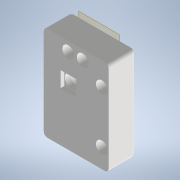
# Autodesk Inventor part: 30_ESP32_Camera_tray
Saved by Autodesk Inventor 2022 (Build 260153000, 153)
## iProperties
Created: 2022-06-11
Part Number: 30_ESP32_Camera_tray
Material: Generisch
Document SubType Name: Modeling
Designer: diederichbenedict
Density: 1 g/cm^3
Appearance: Vorgabe
Author: diederichbenedict
Autodesk Inventor part; units mm, degrees
ref_plane "YZ Plane" through (0, 0, 0) normal (1, 0, 0) x (0, 1, 0)
ref_plane "XZ Plane" through (0, 0, 0) normal (0, 1, 0) x (-1, 0, 0)
ref_plane "XY Plane" through (0, 0, 0) normal (0, 0, 1) x (1, 0, 0)
ref_plane "Arbeitsebene1" through (0, 0, 0) normal (0, 0, 1) x (1, 0, 0)
sketch "Skizze1" plane through (0, 0, 0) normal (0, 0, 1) x (1, 0, 0)
  line L0 (20, 36) -> (0, 36) projected
  line L1 (0, 0) -> (0, 36) projected
  line L2 (20, 0) -> (0, 0) projected
  line L3 (20, 0) -> (20, 36) projected
  arc A0 (15.4309, 14.7711) -> (15.4309, 17.2289) centre (16.1016, 16) ccw projected
  arc A1 (15.4309, 17.2289) -> (15.4309, 14.7711) centre (8.2858, 16) ccw projected
  circle A2 centre (8.2858, 30.7551) radius 1.4 projected
  circle A3 centre (16.1016, 30.7551) radius 1.4 projected
  circle A4 centre (8.2858, 16) radius 6 projected
  line L4 (14.1858, 12.5359) -> (8.3358, 9.1584)
  line L5 (2.3358, 12.6225) -> (2.3358, 19.3775)
  line L6 (8.3358, 22.8416) -> (14.1858, 19.4641)
  circle A5 centre (8.2858, 16) radius 5.95
  arc A6 (14.1858, 12.5359) -> (14.1858, 19.4641) centre (12.1858, 16) ccw
  arc A7 (2.3358, 12.6225) -> (8.3358, 9.1584) centre (6.3358, 12.6225) ccw
  arc A8 (8.3358, 22.8416) -> (2.3358, 19.3775) centre (6.3358, 19.3775) ccw
  line L7 (-5, 36) -> (30, 36)
  line L8 (30, 36) -> (30, -15)
  line L9 (30, -15) -> (-5, -15)
  line L10 (-5, -15) -> (-5, 36)
  point P0 (20.1858, 16)
  point P1 (2.3358, 5.6943)
  point P2 (2.3358, 26.3057)
  point P3 (10.5914, 21.5393)
  point P4 (11.9302, 20.7664)
  point P5 (11.9302, 11.2336)
  point P6 (10.5914, 10.4607)
  point P7 (2.3358, 15.227)
  point P8 (2.3358, 16.773)
  dimension "d0" = 11.9
  dimension "d1" = 4
  dimension "d2" = 10
  dimension "d3" = 0
  dimension "d4" = 5
  dimension "d5" = 15
  constraints: 14 end point, 7 tangent, 6 point on circle, 6 point on line, 4 centre point, 2 coincident, 2 equal radius, 2 parallel, 1 horizontal, 1 perpendicular, 7 other
  measures "d0" diameter of A5
  measures "d1" radius of A6
  measures "d2" distance between parallel lines of L8 L3
  measures "d3" distance between parallel lines of L7 L0
  measures "d4" distance between parallel lines of L1 L10
  measures "d5" distance between parallel lines of L2 L9
extrude "Extrusion1" add sketch "Skizze1" along normal blind 10 contours L3 L2 L1 L0 | L7 L8 L9 L10 L1 L2 L3 | A6 A0 | A1 A7 L4 A4 A6 | A6 L6 A4 A8 A1 | A1 A8 L5 A4 A7
sketch "Skizze2" plane through (0, 0, 10) normal (0, 0, 1) x (1, 0, 0)
  line L0 (-5, -15) -> (30, -15) projected
  line L1 (30, -15) -> (30, 36) projected
  line L2 (30, 36) -> (-5, 36) projected
  line L3 (-5, 36) -> (-5, -15) projected
  circle A0 centre (16.1016, 30.7551) radius 1.4 projected
  circle A1 centre (8.2858, 30.7551) radius 1.4 projected
  arc A2 (8.3358, 22.8416) -> (2.3358, 19.3775) centre (6.3358, 19.3775) ccw projected
  line L4 (8.3358, 22.8416) -> (10.5914, 21.5393) projected
  arc A3 (11.9302, 20.7664) -> (10.5914, 21.5393) centre (8.2858, 16) ccw projected
  line L5 (11.9302, 20.7664) -> (14.1858, 19.4641) projected
  arc A4 (14.1858, 12.5359) -> (14.1858, 19.4641) centre (12.1858, 16) ccw projected
  line L6 (14.1858, 12.5359) -> (11.9302, 11.2336) projected
  arc A5 (10.5914, 10.4607) -> (11.9302, 11.2336) centre (8.2858, 16) ccw projected
  line L7 (10.5914, 10.4607) -> (8.3358, 9.1584) projected
  arc A6 (2.3358, 12.6225) -> (8.3358, 9.1584) centre (6.3358, 12.6225) ccw projected
  line L8 (2.3358, 12.6225) -> (2.3358, 15.227) projected
  arc A7 (2.3358, 16.773) -> (2.3358, 15.227) centre (8.2858, 16) ccw projected
  line L9 (2.3358, 16.773) -> (2.3358, 19.3775) projected
  circle A8 centre (8.2858, 16) radius 3.9
  point P0 (0, 0)
  dimension "d8" = 7.8
  constraints: 1 centre point, 1 coincident
  measures "d8" diameter of A8
extrude "Extrusion2" add sketch "Skizze2" along normal up to surface (2.9472 mm away) contours L3 L2 L1 L0 | L4 A3 L5 A4 L6 A5 L7 A6 L8 A7 L9 A2
sketch "Skizze3" plane through (0, 0, 12.9472) normal (0, 0, 1) x (1, 0, 0)
  circle A0 centre (8.2858, 16) radius 3.6158 projected
  line L0 (4.0358, 12) -> (4.0358, 20) projected
  line L1 (12.5358, 20) -> (12.5358, 12) projected
  line L2 (4.0358, 20.25) -> (12.5358, 20.25)
  line L3 (12.5358, 20.25) -> (12.5358, 11.75)
  line L4 (12.5358, 11.75) -> (4.0358, 11.75)
  line L5 (4.0358, 11.75) -> (4.0358, 20.25)
  line L6 (4.0358, 20.25) -> (12.5358, 11.75) construction
  line L7 (12.5358, 20.25) -> (4.0358, 11.75) construction
  line L8 (30, -15) -> (30, 36) projected
  line L9 (30, 36) -> (-5, 36) projected
  line L10 (-5, 36) -> (-5, -15) projected
  line L11 (-5, -15) -> (30, -15) projected
  circle A1 centre (8.2858, 16) radius 3.9 projected
  circle A2 centre (8.2858, 30.7551) radius 1.4 projected
  circle A3 centre (16.1016, 30.7551) radius 1.4 projected
  point P0 (0, 0)
  point P1 (11.389, 20.2649)
  dimension "d11" = 8.5
  dimension "d12" = 8.5
  constraints: 12 end point, 2 midpoint, 2 parallel, 1 horizontal, 1 perpendicular, 1 other
  measures "d11" distance of L3.end L4.end
  measures "d12" distance of L2.end L3.end
extrude "Extrusion3" add sketch "Skizze3" along normal blind 2 contours L11 L10 L9 L8 | A3
sketch "Skizze4" plane through (0, 0, 14.9472) normal (0, 0, 1) x (1, 0, 0)
  circle A0 centre (8.2858, 30.7551) radius 1.4 projected
  circle A1 centre (16.1016, 30.7551) radius 1.4 projected
  arc A2 (21.7732, 26.3966) -> (20.7732, 27.3966) centre (20.7732, 26.3966) ccw projected
  arc A3 (20.7732, -12.6034) -> (21.7732, -11.6034) centre (20.7732, -11.6034) ccw projected
  circle A4 centre (26.449, 23.3562) radius 1.4
  circle A5 centre (26.449, -4.8113) radius 1.4
  point P0 (0, 0)
  dimension "d23" = 2.8
  dimension "d24" = 2.8
  constraints: 2 centre point
  measures "d23" diameter of A4
  measures "d24" diameter of A5
hole "Bohrung1" at (8.2858, 30.7551, 14.9472) at (16.1016, 30.7551, 14.9472) at (26.449, 23.3562, 14.9472) at (26.449, -4.8113, 14.9472) direction (0, 0, -1) diameter 2.8 depth 30 counterbore diameter 6.5 counterbore depth 12
fillet "Rundung1" radius 2 8 edges at (-5, -15, 7.4736) (-5, 36, 7.4736) (30, 36, 7.4736) (30, 10.5, 0) (12.5, -15, 0) (-5, 10.5, 0) (12.5, 36, 0) (30, -15, 7.4736)
